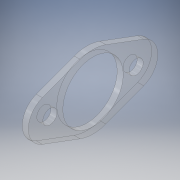
# Autodesk Inventor part: Ball Bearing Ends
Saved by Autodesk Inventor 2017 (Build 210142000, 142)
## iProperties
Created: 2018-05-11
Part Number: Ball Bearing Ends
Material: Polycarbonate, Clear
Document SubType Name: Modeling
Designer: Steven
Density: 1.2 g/cm^3
Appearance: Polycarbonate - Clear
Author: Steven
Autodesk Inventor part; units mm, degrees
ref_plane "YZ Plane" through (0, 0, 0) normal (1, 0, 0) x (0, 1, 0)
ref_plane "XZ Plane" through (0, 0, 0) normal (0, 1, 0) x (-1, 0, 0)
ref_plane "XY Plane" through (0, 0, 0) normal (0, 0, 1) x (1, 0, 0)
sketch "Sketch1" plane through (0, 0, 0) normal (1, 0, 0) x (0, 1, 0)
  circle A0 centre (0, 0) radius 8.89
  circle A1 centre (0, 0) radius 10.795 construction
  line L0 (0, 0) -> (0, 12.7)
  line L1 (0, 0) -> (0, -12.7)
  circle A2 centre (0, -12.7) radius 2.0955
  circle A3 centre (0, 12.7) radius 2.0955
  circle A4 centre (0, 12.7) radius 6.35 construction
  circle A5 centre (0, -12.7) radius 6.35 construction
  line L2 (5.9484, 14.9225) -> (10.1122, 3.7782)
  line L3 (10.1122, -3.7783) -> (5.9484, -14.9225)
  line L4 (-5.9484, -14.9225) -> (-10.1122, -3.7782)
  line L5 (-5.9484, 14.9225) -> (-10.1122, 3.7782)
  arc A6 (5.9484, 14.9225) -> (-5.9484, 14.9225) centre (0, 12.7) ccw
  arc A7 (10.1122, -3.7783) -> (10.1122, 3.7782) centre (0, 0) ccw
  arc A8 (-5.9484, -14.9225) -> (5.9484, -14.9225) centre (0, -12.7) ccw
  arc A9 (-10.1122, 3.7782) -> (-10.1122, -3.7782) centre (0, 0) ccw
  dimension "d0" = 17.78
  dimension "d1" = 21.59
  dimension "d2" = 12.7
  dimension "d3" = 12.7
  dimension "d4" = 4.191
  dimension "d5" = 4.191
  dimension "d6" = 12.7
  dimension "d7" = 12.7
  constraints: 16 point on circle, 14 tangent, 12 end point, 10 centre point, 6 coincident, 2 concentric, 2 vertical
  measures "d0" diameter of A0
  measures "d1" diameter of A1
  measures "d2" distance of L0.start L0.end
  measures "d3" distance of L0.start L1.end
  measures "d4" diameter of A2
  measures "d5" diameter of A3
  measures "d6" diameter of A4
  measures "d7" diameter of A5
extrude "Extrusion1" add sketch "Sketch1" along normal blind 1.778
body "Solid1"
